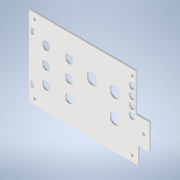
# Autodesk Inventor part: Steckerplatte1
Saved by Autodesk Inventor 2022 (Build 260153000, 153)
## iProperties
Created: 2022-02-01
Part Number: Steckerplatte1
Material: Generic
Document SubType Name: Modeling
Designer: Fabijansven
Density: 1 g/cm^3
Appearance: Default
Author: Fabijansven
Autodesk Inventor part; units mm, degrees
ref_plane "YZ Plane" through (0, 0, 0) normal (1, 0, 0) x (0, 1, 0)
ref_plane "XZ Plane" through (0, 0, 0) normal (0, 1, 0) x (-1, 0, 0)
ref_plane "XY Plane" through (0, 0, 0) normal (0, 0, 1) x (1, 0, 0)
sketch "Sketch1" plane through (0, 0, 0) normal (0, 0, 1) x (1, 0, 0)
  line L0 (0, 0) -> (190, 0)
  line L1 (0, 140) -> (0, 0)
  line L2 (190, 0) -> (190, 30)
  line L3 (190, 30) -> (210, 30)
  line L4 (210, 30) -> (210, 74.5)
  line L5 (186, 140) -> (186, 74.5)
  line L6 (186, 74.5) -> (210, 74.5)
  line L7 (186, 140) -> (0, 140)
  dimension "d2" = 20
  dimension "d3" = 30
  dimension "d4" = 140
  dimension "d49" = 24
  dimension "d50" = 65.5
  dimension "d51" = 210
  constraints: 16 end point, 2 horizontal, 2 parallel, 1 perpendicular, 1 vertical
  measures "d2" distance of L2.end L3.end
  measures "d3" distance of L0.end L2.end
  measures "d4" distance of L1.start L0.start
  measures "d49" distance between parallel lines of L4 L5
  measures "d50" distance between parallel lines of L7 L6
  measures "d51" distance between parallel lines of L1 L4
extrude "Extrusion1" add sketch "Sketch1" along normal blind 3
sketch "Sketch2" plane through (0, 0, 3) normal (0, 0, 1) x (1, 0, 0)
  arc A0 (141.1, 85.2251) -> (158.9, 85.2251) centre (150, 90) ccw
  line L0 (210, 30) -> (210, 74.5) projected
  line L1 (250, 140) -> (0, 140) projected
  line L2 (141.1, 94.7749) -> (141.1, 85.2251)
  line L3 (158.9, 94.7749) -> (158.9, 85.2251)
  arc A1 (158.9, 94.7749) -> (141.1, 94.7749) centre (150, 90) ccw
  circle A2 centre (180, 114) radius 6
  line L4 (158.9, 54.7749) -> (158.9, 45.2251)
  arc A3 (158.9, 54.7749) -> (141.1, 54.7749) centre (150, 50) ccw
  line L5 (141.1, 54.7749) -> (141.1, 45.2251)
  arc A4 (141.1, 45.2251) -> (158.9, 45.2251) centre (150, 50) ccw
  arc A5 (101.1, 85.2251) -> (118.9, 85.2251) centre (110, 90) ccw
  arc A6 (118.9, 94.7749) -> (101.1, 94.7749) centre (110, 90) ccw
  line L6 (118.9, 94.7749) -> (118.9, 85.2251)
  line L7 (101.1, 94.7749) -> (101.1, 85.2251)
  arc A7 (63.25, 96.4) -> (76.75, 96.4) centre (70, 100) ccw
  line L8 (63.25, 103.6) -> (63.25, 96.4)
  line L9 (76.75, 103.6) -> (76.75, 96.4)
  arc A8 (76.75, 103.6) -> (63.25, 103.6) centre (70, 100) ccw
  line L10 (76.75, 73.6) -> (76.75, 66.4)
  arc A9 (63.25, 66.4) -> (76.75, 66.4) centre (70, 70) ccw
  line L11 (63.25, 73.6) -> (63.25, 66.4)
  arc A10 (76.75, 73.6) -> (63.25, 73.6) centre (70, 70) ccw
  line L12 (76.75, 43.6) -> (76.75, 36.4)
  arc A11 (63.25, 36.4) -> (76.75, 36.4) centre (70, 40) ccw
  line L13 (63.25, 43.6) -> (63.25, 36.4)
  arc A12 (76.75, 43.6) -> (63.25, 43.6) centre (70, 40) ccw
  line L14 (36.75, 103.6) -> (36.75, 96.4)
  arc A13 (23.25, 96.4) -> (36.75, 96.4) centre (30, 100) ccw
  line L15 (23.25, 103.6) -> (23.25, 96.4)
  arc A14 (36.75, 103.6) -> (23.25, 103.6) centre (30, 100) ccw
  line L16 (36.75, 73.6) -> (36.75, 66.4)
  arc A15 (23.25, 66.4) -> (36.75, 66.4) centre (30, 70) ccw
  line L17 (23.25, 73.6) -> (23.25, 66.4)
  arc A16 (36.75, 73.6) -> (23.25, 73.6) centre (30, 70) ccw
  line L18 (36.75, 43.6) -> (36.75, 36.4)
  arc A17 (23.25, 36.4) -> (36.75, 36.4) centre (30, 40) ccw
  line L19 (23.25, 43.6) -> (23.25, 36.4)
  arc A18 (36.75, 43.6) -> (23.25, 43.6) centre (30, 40) ccw
  circle A19 centre (180, 99) radius 6
  circle A20 centre (180, 84) radius 6
  circle A21 centre (180, 69) radius 6
  point P0 (0, 0)
  dimension "d8" = 60
  dimension "d10" = 17.8
  dimension "d11" = 8.9
  dimension "d12" = 10.1
  dimension "d21" = 12
  dimension "d23" = 30
  dimension "d52" = 26
  dimension "d53" = 50
  dimension "d83" = 40
  dimension "d93" = 40
  dimension "d98" = 40
  dimension "d99" = 40
  dimension "d100" = 13.5
  dimension "d101" = 6.75
  dimension "d102" = 7.65
  dimension "d105" = 30
  dimension "d108" = 40
  dimension "d113" = 15
  constraints: 45 point on circle, 36 end point, 22 centre point, 18 vertical alignment, 9 equal radius, 6 collinear, 2 horizontal, 2 parallel, 2 vertical, 37 other
  measures "d10" distance between parallel lines of L3 L2
  measures "d11" distance from line of L2 A0.centre
  measures "d12" radius of A1
  measures "d21" diameter of A2
  measures "d52" distance from line of L1 A2.centre
  measures "d53" distance from line of L1 A0.centre
  measures "d83" distance of L3.start L4.start
  measures "d93" distance of A0.centre A5.centre
  measures "d98" horizontal distance of A7.centre A5.centre
  measures "d99" distance from line of A7.centre L1
  measures "d100" distance between parallel lines of L8 L9
  measures "d101" distance from line of L8 A7.centre
  measures "d102" radius of A8
  measures "d105" distance of L9.end L10.end
  measures "d108" distance of L9.end L14.end
  measures "d113" distance of A2.centre A19.centre
extrude "Extrusion2" cut sketch "Sketch2" against normal blind 12
sketch "Sketch3" plane through (0, 0, 3) normal (0, 0, 1) x (1, 0, 0)
  circle A0 centre (10, 10) radius 2.75
  circle A1 centre (10, 130) radius 2.75
  circle A2 centre (180, 130) radius 2.75
  circle A3 centre (180, 10) radius 2.75
  circle A4 centre (200, 52) radius 2.75
  line L0 (0, 140) -> (0, 0) projected
  line L1 (186, 140) -> (0, 140) projected
  line L2 (0, 0) -> (190, 0) projected
  line L3 (190, 0) -> (190, 30) projected
  line L4 (210, 30) -> (210, 74.5) projected
  line L5 (190, 30) -> (210, 30) projected
  dimension "d54" = 10
  dimension "d55" = 10
  dimension "d56" = 5.5
  dimension "d57" = 10
  dimension "d58" = 10
  dimension "d59" = 5.5
  dimension "d60" = 10
  dimension "d61" = 10
  dimension "d62" = 5.5
  dimension "d63" = 10
  dimension "d64" = 22
  dimension "d65" = 5.5
  dimension "d67" = 10
  dimension "d68" = 10
  dimension "d69" = 5.5
  constraints: 5 centre point
  measures "d54" distance from line of L0 A1.centre
  measures "d55" distance from line of A1.centre L1
  measures "d56" diameter of A1
  measures "d57" distance from line of L0 A0.centre
  measures "d58" distance from line of L2 A0.centre
  measures "d59" diameter of A0
  measures "d60" distance from line of L2 A3.centre
  measures "d61" distance from line of L3 A3.centre
  measures "d62" diameter of A3
  measures "d63" distance from line of L4 A4.centre
  measures "d64" distance from line of L5 A4.centre
  measures "d65" diameter of A4
  measures "d67" distance from line of L3 A2.centre
  measures "d68" distance from line of L1 A2.centre
  measures "d69" diameter of A2
extrude "Holes" cut sketch "Sketch3" against normal blind 12
sketch "Sketch4" plane through (0, 0, 3) normal (0, 0, 1) x (1, 0, 0)
  line L0 (3, 115) -> (8.2, 115)
  line L1 (8.2, 115) -> (8.2, 104.8)
  line L2 (8.2, 104.8) -> (3, 104.8)
  line L3 (3, 104.8) -> (3, 115)
  line L4 (3, 35.2) -> (8.2, 35.2)
  line L5 (8.2, 35.2) -> (8.2, 25)
  line L6 (8.2, 25) -> (3, 25)
  line L7 (3, 25) -> (3, 35.2)
  line L8 (0, 140) -> (0, 0) projected
  line L9 (0, 0) -> (190, 0) projected
  line L10 (186, 140) -> (0, 140) projected
  dimension "d72" = 3
  dimension "d73" = 3
  dimension "d74" = 25
  dimension "d75" = 25
  dimension "d76" = 10.2
  dimension "d77" = 5.2
  dimension "d78" = 10.2
  constraints: 16 end point, 4 parallel, 2 horizontal, 2 perpendicular, 1 point on line
  measures "d72" distance between parallel lines of L8 L3
  measures "d73" distance between parallel lines of L8 L7
  measures "d74" distance between parallel lines of L9 L6
  measures "d75" distance from line of L0.start L10
  measures "d76" distance of L0.end L1.end
  measures "d77" distance between parallel lines of L3 L1
  measures "d78" distance of L4.end L5.end
extrude "Extrusion4" cut sketch "Sketch4" against normal blind 12
equation "\"d45\" = d26"
equation "\"d58\" = d54"
equation "\"d59\" = d56"
equation "\"d60\" = d54"
equation "\"d61\" = d54"
equation "\"d62\" = d56"
equation "\"d63\" = d54"
equation "\"d65\" = d56"
equation "\"d70\" = d26"
equation "\"d79\" = d26"
equation "\"d26\" = 12"
body "Solid1"
